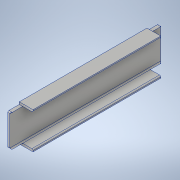
# Autodesk Inventor part: NASA-20-FR-FP-01
Saved by Autodesk Inventor 2020 (Build 240168000, 168)
## iProperties
Created: 2019-09-05
Part Number: NASA-20-FR-FP-01
Material: Aluminum 6061
Description: FRONT PLATE
Document SubType Name: Modeling
Designer: Rick Szalay
Stock Number: 1630T31
Density: 2.7 g/cm^3
Appearance: Aluminum - Flat
Author: Rick Szalay
Autodesk Inventor part; units mm, degrees
ref_plane "YZ Plane" through (0, 0, 0) normal (1, 0, 0) x (0, 1, 0)
ref_plane "XZ Plane" through (0, 0, 0) normal (0, 1, 0) x (-1, 0, 0)
ref_plane "XY Plane" through (0, 0, 0) normal (0, 0, 1) x (1, 0, 0)
sketch "Sketch3" plane through (0, 0, 0) normal (0, 0, 1) x (1, 0, 0)
  line L0 (0, 25.4) -> (0, -25.4)
  line L1 (0, 25.4) -> (19.05, 25.4)
  line L2 (19.05, 25.4) -> (19.05, 22.225)
  line L3 (19.05, 22.225) -> (3.048, 22.225)
  line L4 (3.048, 22.225) -> (3.048, -22.225)
  line L5 (3.048, -22.225) -> (19.05, -22.225)
  line L6 (19.05, -22.225) -> (19.05, -25.4)
  line L7 (19.05, -25.4) -> (0, -25.4)
  line L8 (0, 0) -> (3.048, 0) construction
  dimension "d7" = 50.8
  dimension "d19" = 16.002
  dimension "d20" = 19.05
  dimension "d21" = 3.175
  constraints: 18 end point, 6 perpendicular, 2 horizontal, 2 midpoint, 1 coincident, 1 vertical, 1 other
  measures "d7" distance of L0.start L0.end
  measures "d19" distance between parallel lines of L2 L4
  measures "d20" distance between parallel lines of L6 L0
  measures "d21" distance between parallel lines of L3 L1
extrude "Extrusion3" add sketch "Sketch3" along normal mid plane 209.296
fillet "Fillet1" radius 1.5875 4 edges at (19.05, 22.225, 0) (19.05, -22.225, 0) (3.048, -22.225, 0) (3.048, 22.225, 0)
sketch "Sketch4" plane through (0, -25.4, 104.648) normal (-1, 0, 0) x (0, 0, 1)
  line L0 (0, 50.8) -> (-209.296, 50.8) projected
  line L1 (-209.296, 50.8) -> (-193.294, 50.8)
  line L2 (-193.294, 50.8) -> (-193.294, 47.625)
  line L3 (-193.294, 47.625) -> (-209.296, 47.625)
  line L4 (-209.296, 47.625) -> (-209.296, 50.8)
  line L5 (0, 46.0375) -> (-209.296, 46.0375) projected
  line L6 (-209.296, 4.7625) -> (0, 4.7625) projected
  line L7 (-209.296, 0) -> (0, 0) projected
  line L8 (-209.296, 0) -> (0, 0) projected
  line L9 (-209.296, 0) -> (-193.294, 0)
  line L10 (-193.294, 0) -> (-193.294, 3.175)
  line L11 (-193.294, 3.175) -> (-209.296, 3.175)
  line L12 (-209.296, 3.175) -> (-209.296, 0)
  line L13 (0, 3.175) -> (-209.296, 3.175) projected
  line L14 (-209.296, 47.625) -> (0, 47.625) projected
  point P0 (-104.648, 25.4)
  dimension "d14" = 16.002
  constraints: 16 end point, 4 parallel, 3 collinear, 2 horizontal, 2 perpendicular
  measures "d14" distance between parallel lines of L4 L2
extrude "Extrusion4" cut sketch "Sketch4" against normal through all
mirror "Mirror1" about plane through (0, 0, 0) normal (0, 0, 1) of "Extrusion4"
fillet "Fillet3" radius 1.5875 4 edges at (2.3177, 22.225, -104.648) (2.3177, -22.225, -104.648) (2.3177, 22.225, 104.648) (2.3177, -22.225, 104.648)
equation "\"d11\" = Length"
equation "\"Length\" = 209.296"
body "Solid2"
